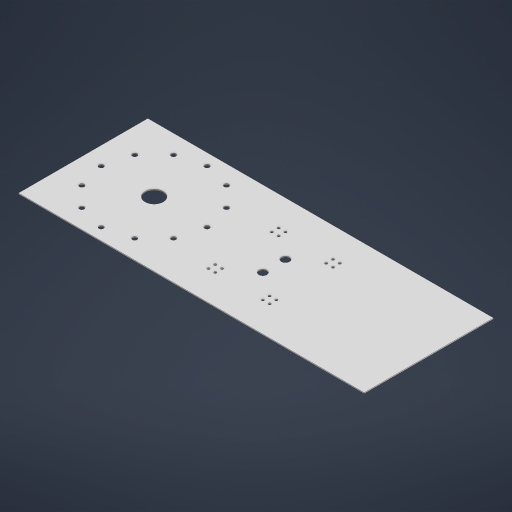
# Autodesk Inventor part: ChassisTop V2
Saved by Autodesk Inventor 2024 (Build 280153000, 153)
## iProperties
Created: 2023-10-24
Part Number: ChassisTop V2
Material: Generic
Document SubType Name: Modeling
Designer: avsar
Density: 1 g/cm^3
Appearance: Default
Author: avsar
Autodesk Inventor part; units mm, degrees
ref_plane "YZ Plane" through (0, 0, 0) normal (1, 0, 0) x (0, 1, 0)
ref_plane "XZ Plane" through (0, 0, 0) normal (0, 1, 0) x (-1, 0, 0)
ref_plane "XY Plane" through (0, 0, 0) normal (0, 0, 1) x (1, 0, 0)
sketch "Sketch1" plane through (0, 0, 0) normal (0, 1, 0) x (-1, 0, 0)
  line L0 (-305.435, 114.3) -> (305.435, 114.3)
  line L1 (305.435, 114.3) -> (305.435, -114.3)
  line L2 (305.435, -114.3) -> (-305.435, -114.3)
  line L3 (-305.435, -114.3) -> (-305.435, 114.3)
  line L4 (-305.435, 114.3) -> (305.435, -114.3) construction
  line L5 (305.435, 114.3) -> (-305.435, -114.3) construction
  point P0 (0, 0)
  dimension "d0" = 610.87
  dimension "d1" = 228.6
  constraints: 12 end point, 2 midpoint, 2 parallel, 1 horizontal, 1 perpendicular
  measures "d0" distance of L1.end L2.end
  measures "d1" distance of L0.end L1.end
extrude "Extrusion1" add sketch "Sketch1" along normal blind 1.5875
sketch "Sketch3" plane through (0, 1.5875, 0) normal (0, 1, 0) x (1, 0, 0)
  circle A0 centre (-180, 0) radius 93.5 construction
  circle A1 centre (-180, 93.5) radius 4
  circle A2 centre (-226.75, 80.9734) radius 4
  circle A3 centre (-260.9734, 46.75) radius 4
  circle A4 centre (-273.5, 0) radius 4
  circle A5 centre (-260.9734, -46.75) radius 4
  circle A6 centre (-226.75, -80.9734) radius 4
  circle A7 centre (-180, -93.5) radius 4
  circle A8 centre (-133.25, -80.9734) radius 4
  circle A9 centre (-99.0266, -46.75) radius 4
  circle A10 centre (-86.5, 0) radius 4
  circle A11 centre (-99.0266, 46.75) radius 4
  circle A12 centre (-133.25, 80.9734) radius 4
  circle A13 centre (-180, 0) radius 16
  point P0 (0, 0)
  dimension "d5" = 187
  dimension "d6" = 180
  dimension "d7" = 8
  dimension "d10" = 360
  dimension "d12" = 32
  constraints: 13 centre point, 2 vertical alignment, 1 coincident, 1 horizontal alignment, 27 other
  measures "d6" distance of point (0, 0) point (-180, 0)
  measures "d7" diameter of A1
  measures "d12" diameter of A13
extrude "Extrusion2" cut sketch "Sketch3" against normal through all
sketch "Sketch4" plane through (0, 1.5875, 0) normal (0, 1, 0) x (1, 0, 0)
  circle A0 centre (-180, 0) radius 16 construction
  circle A1 centre (32, 0) radius 7 construction
  circle A2 centre (-16, 56) radius 2.5 construction
  circle A3 centre (-22, 62) radius 2
  circle A4 centre (-22, 50) radius 2
  circle A5 centre (-10, 50) radius 2
  circle A6 centre (-10, 62) radius 2
  line L0 (32, 7) -> (32, -7) construction
  line L1 (25, 0) -> (39, 0) construction
  circle A7 centre (86, 62) radius 2
  circle A8 centre (86, 50) radius 2
  circle A9 centre (74, 50) radius 2
  circle A10 centre (74, 62) radius 2
  circle A11 centre (-22, -62) radius 2
  circle A12 centre (-22, -50) radius 2
  circle A13 centre (-10, -50) radius 2
  circle A14 centre (-10, -62) radius 2
  circle A15 centre (86, -62) radius 2
  circle A16 centre (86, -50) radius 2
  circle A17 centre (74, -50) radius 2
  circle A18 centre (74, -62) radius 2
  circle A19 centre (32, -20) radius 7
  circle A20 centre (32, 20) radius 7
  point P0 (0, 0)
  dimension "d22" = 14
  dimension "d23" = 212
  dimension "d24" = 5
  dimension "d25" = 48
  dimension "d26" = 56
  dimension "d27" = 4
  dimension "d28" = 6
  dimension "d29" = 6
  dimension "d34" = 360
  dimension "d36" = 14
  dimension "d37" = 20
  dimension "d38" = 14
  dimension "d39" = 20
  constraints: 20 centre point, 12 symmetric about line, 4 end point, 4 point on circle, 2 midpoint, 2 vertical alignment, 1 coincident, 1 horizontal, 1 horizontal alignment, 1 vertical, 21 other
  measures "d22" diameter of A1
  measures "d23" distance of A1.centre A0.centre
  measures "d24" diameter of A2
  measures "d25" horizontal distance of A1.centre A2.centre
  measures "d26" vertical distance of A2.centre A1.centre
  measures "d27" diameter of A3
  measures "d28" horizontal distance of A2.centre A3.centre
  measures "d29" horizontal distance of A2.centre A3.centre
  measures "d36" diameter of A19
  measures "d37" distance of A19.centre A1.centre
  measures "d38" diameter of A20
  measures "d39" distance of A20.centre A1.centre
extrude "Extrusion3" cut sketch "Sketch4" against normal through all
body "Solid1"
